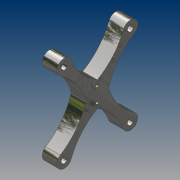
# Autodesk Inventor part: 21_Tam_go_trung_gian
Saved by Autodesk Inventor 2021 (Build 250183000, 183)
## iProperties
Created: 2024-04-07
Part Number: 21_Tam_go_trung_gian
Material: Stainless Steel, Austenitic
Document SubType Name: Modeling
Designer: Admin
Density: 8 g/cm^3
Appearance: Semi-Polished
Author: Admin
Autodesk Inventor part; units mm, degrees
ref_plane "YZ Plane" through (0, 0, 0) normal (1, 0, 0) x (0, 1, 0)
ref_plane "XZ Plane" through (0, 0, 0) normal (0, 1, 0) x (-1, 0, 0)
ref_plane "XY Plane" through (0, 0, 0) normal (0, 0, 1) x (1, 0, 0)
sketch "Sketch1" plane through (0, 0, 0) normal (1, 0, 0) x (0, 1, 0)
  line L0 (-27.5, 22.5) -> (27.5, 22.5)
  line L1 (27.5, 22.5) -> (27.5, -22.5)
  line L2 (27.5, -22.5) -> (-27.5, -22.5)
  line L3 (-27.5, -22.5) -> (-27.5, 22.5)
  line L4 (-27.5, 22.5) -> (27.5, -22.5) construction
  line L5 (27.5, 22.5) -> (-27.5, -22.5) construction
  circle A0 centre (27.5, 22.5) radius 5
  circle A1 centre (27.5, -22.5) radius 5
  line L6 (0, -22.5) -> (0, 22.5) construction
  circle A2 centre (0, 0) radius 7.5
  arc A3 (29.2912, 17.8319) -> (6.8009, -3.1619) centre (43.9793, -20.4469) ccw
  arc A4 (-1.7526, 7.2924) -> (23.279, 25.1801) centre (-11.3332, 47.1573) ccw
  line L7 (27.5, 0) -> (-27.5, 0) construction
  arc A5 (6.8009, 3.1619) -> (29.2912, -17.8319) centre (43.9793, 20.4469) ccw
  arc A6 (23.279, -25.1801) -> (-1.7526, -7.2924) centre (-11.3332, -47.1573) ccw
  circle A7 centre (-27.5, 22.5) radius 5
  circle A8 centre (-27.5, -22.5) radius 5
  arc A9 (-6.8009, -3.1619) -> (-29.2912, 17.8319) centre (-43.9793, -20.4469) ccw
  arc A10 (-23.279, 25.1801) -> (1.7526, 7.2924) centre (11.3332, 47.1573) ccw
  arc A11 (-29.2912, -17.8319) -> (-6.8009, 3.1619) centre (-43.9793, 20.4469) ccw
  arc A12 (1.7526, -7.2924) -> (-23.279, -25.1801) centre (11.3332, -47.1573) ccw
  point P0 (23.279, 25.1801)
  point P1 (0, 7.7548)
  point P2 (-23.279, 25.1801)
  point P3 (-8.4416, 0)
  point P4 (-29.2912, -17.8319)
  point P5 (-23.279, -25.1801)
  point P6 (0, -7.7548)
  point P7 (23.279, -25.1801)
  point P8 (29.2912, -17.8319)
  point P9 (8.4416, 0)
  dimension "d3" = 15
  dimension "d0" = 55
  dimension "d1" = 45
  dimension "d2" = 10
  dimension "d4" = 41
  constraints: 23 symmetric about line, 16 end point, 16 point on circle, 10 centre point, 6 midpoint, 3 coincident, 2 parallel, 1 horizontal, 1 perpendicular, 1 vertical, 20 other
  measures "d0" distance of L1.end L2.end
  measures "d1" distance of L0.end L1.end
  measures "d2" diameter of A1
  measures "d4" radius of A3
extrude "Extrusion1" add sketch "Sketch1" along normal blind 10 contours L3 A7 L0 | L0 A7 L3 | A7 A10 L0 | L0 A10 A4 A2 A11 A9 L3 A7 | L3 A9 A7 | A4 A0 L0 | L0 A0 L1 A3 A5 A2 A10 A4 | A10 A2 A4 | A11 A9 A2 A6 A12 L2 A8 L3 | L3 A8 A11 | A11 A2 A9 | A0 L1 L0 | L0 L1 A0 | A2 | A8 L2 L3 | L3 L2 A8 | A0 A3 L1 | A5 A3 A2 | L2 A12 A8 | A2 A12 A6 | A5 L1 A1 L2 A6 A12 A2 A3 | A5 A1 L1 | L2 A1 A6 | A1 L2 L1 | L1 L2 A1
sketch "Sketch2" plane through (10, 0, 0) normal (1, 0, 0) x (0, 0, -1)
  arc A0 (-25.1801, -23.279) -> (-7.7548, 0) centre (-47.1573, 11.3332) ccw projected
  arc A1 (-25.1801, -23.279) -> (-17.8319, -29.2912) centre (-22.5, -27.5) ccw projected
  arc A2 (0, -8.4416) -> (-17.8319, -29.2912) centre (20.4469, -43.9793) ccw projected
  arc A3 (17.8319, -29.2912) -> (0, -8.4416) centre (-20.4469, -43.9793) ccw projected
  arc A4 (17.8319, -29.2912) -> (25.1801, -23.279) centre (22.5, -27.5) ccw projected
  arc A5 (7.7548, 0) -> (25.1801, -23.279) centre (47.1573, 11.3332) ccw projected
  arc A6 (25.1801, 23.279) -> (7.7548, 0) centre (47.1573, -11.3332) ccw projected
  arc A7 (25.1801, 23.279) -> (17.8319, 29.2912) centre (22.5, 27.5) ccw projected
  arc A8 (0, 8.4416) -> (17.8319, 29.2912) centre (-20.4469, 43.9793) ccw projected
  arc A9 (-17.8319, 29.2912) -> (0, 8.4416) centre (20.4469, 43.9793) ccw projected
  arc A10 (-17.8319, 29.2912) -> (-25.1801, 23.279) centre (-22.5, 27.5) ccw projected
  arc A11 (-7.7548, 0) -> (-25.1801, 23.279) centre (-47.1573, -11.3332) ccw projected
  point P0 (0, 0)
hole "Hole1" at (10, 27.5, 22.5) at (10, -27.5, 22.5) at (10, -27.5, -22.5) at (10, 27.5, -22.5) direction (-1, 0, 0) diameter 4.2 end through all
sketch "Sketch3" plane through (0, 0, 0) normal (-1, 0, 0) x (0, 0, 1)
  line L0 (0, 5) -> (0, -5)
  line L1 (0, 0) -> (4.5458, 0) construction
  dimension "d14" = 10
  constraints: 4 end point, 1 horizontal, 1 symmetric about line, 1 vertical
  measures "d14" distance of L0.start L0.end
hole "Hole2" at (0, 5, 0) at (0, -5, 0) direction (1, 0, 0) diameter 1.8 end through all
body "Solid1"
